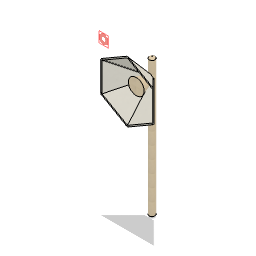
Sarah_meylan (Autodesk Fusion 360 design; units mm, degrees)
Autodesk Fusion 360 part; units mm, degrees
sketch "Esquisse1" plane through (0, 0, 0) normal (0, 1, 0) x (1, 0, 0)
  circle A0 centre (0, 0) radius 16.5
  dimension "d1" = 33
  constraint coincident A0.centre origin
  measures "d1" diameter of A0
extrude "Extrusion1" add sketch "Esquisse1" along normal blind 770 makes body 1
sketch "Esquisse3" plane through (0, 0, 0) normal (0, 1, 0) x (1, 0, 0)
  circle A0 centre (0, 0) radius 14
  dimension "d5" = 28
  constraint coincident A0.centre origin
  measures "d5" diameter of A0
extrude "Extrusion2" cut sketch "Esquisse3" along normal blind 770 bodies 1
sketch "Esquisse4" plane through (0, 0, 0) normal (0, 1, 0) x (1, 0, 0)
  circle A0 centre (0, 0) radius 16.5
  dimension "d8" = 33
  constraint coincident A0.centre origin
  measures "d8" diameter of A0
extrude "Extrusion3" add sketch "Esquisse4" against normal blind 10 separate body makes body 2
fillet "Congé1" radius 15 1 edges at (-15.3834, -10, -5.9667) on bodies 2
sketch "Esquisse6" plane through (0, 0, 0) normal (0, 0, 1) x (1, 0, 0)
sketch "Esquisse7" plane through (0, 0, 0) normal (0, 0, 1) x (1, 0, 0)
  line L0 (-275, 755) -> (-250, 740)
  line L1 (-250, 740) -> (-250, 710)
  line L2 (-250, 710) -> (-275, 695)
  line L3 (-275, 695) -> (-301.8648, 710)
  line L4 (-301.8648, 710) -> (-301.8648, 740)
  line L5 (-301.8648, 740) -> (-275, 755)
  constraint vertical L1
  constraint parallel L1 L4
sketch "Esquisse8" plane through (0, 0, 0) normal (0, 0, 1) x (1, 0, 0)
  line L0 (-275.4763, 755.2472) -> (-302.1986, 739.7984)
  line L1 (-302.1986, 739.7984) -> (-302.1986, 710)
  line L2 (-302.1986, 710) -> (-275.4763, 694.7044)
  line L3 (-275.4763, 694.7044) -> (-249.0191, 710)
  line L4 (-249.0191, 710) -> (-249.0191, 740)
  line L5 (-249.0191, 740) -> (-275.4763, 755.2472)
  constraint vertical L1
  constraint parallel L0 L3
  constraint parallel L1 L4
extrude "Extrusion5" add sketch "Esquisse8" along normal blind 125 draft 45 separate body makes body 3
move_body "Déplacer1" bodies 3 to x (1, 0, 0) y (0, 1, 0) z (0, 0, 1) at (275, -50, 15)
shell "Coque1" thickness 5 removed faces 1 at (-50.9798, 703.9976, 140) on bodies 3
fillet "Congé2" radius 15 tangency weight 2 6 edges at (88.4809, 726.1173, 77.5) (-0.5257, 777.4116, 77.5) (88.4809, 623.9398, 77.5) (-89.6986, 725.8586, 77.5) (-89.6986, 623.7601, 77.5) (-0.3209, 572.6013, 77.5) on bodies 3
sketch "Esquisse9" plane through (0, 0, 20) normal (0, 0, 1) x (1, 0, 0)
  line L0 (23.9099, 688.8032) -> (-0.4746, 702.8559)
  line L1 (-0.4746, 702.8559) -> (-25.1275, 688.6034)
  line L2 (-25.1275, 688.6034) -> (-25.1275, 661.2009)
  line L3 (-25.1275, 661.2009) -> (-0.4814, 647.0937)
  line L4 (-0.4814, 647.0937) -> (23.9099, 661.1949)
  line L5 (23.9099, 661.1949) -> (23.9099, 688.8032)
  circle A0 centre (0.3686, 674.9991) radius 22.5
  dimension "d21" = 45
  measures "d21" diameter of A0
sketch "Esquisse10" plane through (0, 0, 20) normal (0, 0, 1) x (1, 0, 0)
  line L0 (23.9099, 688.8032) -> (-0.4746, 702.8559)
  line L1 (-0.4746, 702.8559) -> (-25.1275, 688.6034)
  line L2 (-25.1275, 688.6034) -> (-25.1275, 661.2009)
  line L3 (-25.1275, 661.2009) -> (-0.4814, 647.0937)
  line L4 (-0.4814, 647.0937) -> (23.9099, 661.1949)
  line L5 (23.9099, 661.1949) -> (23.9099, 688.8032)
  circle A0 through (44.9296, 674.9991, 70) (-22.5704, 713.9702, 70) (-22.5704, 636.0279, 70)
  dimension "d24" = 90
extrude "Extrusion7" add sketch "Esquisse10" against normal blind 70 draft -20 contours A0 in plane through (0, 0, 90) normal (0, 0, 1) bodies 3
sketch "Esquisse15" plane through (0, 0, 0) normal (0, 1, 0) x (1, 0, 0)
  circle A0 centre (125, 0) radius 16.5
  dimension "d31" = 33
  measures "d31" diameter of A0
extrude "Extrusion8" add sketch "Esquisse15" along normal blind 10 separate body makes body 4
move_body "Déplacer2" bodies 4 to x (1, 0, 0) y (0, 1, 0) z (0, 0, 1) at (-125, 770, 0)
fillet "Congé3" radius 15 1 faces at (-0.411, 780, -5.2396) on bodies 4
sketch "Esquisse14" plane through (0, 0, 0) normal (0, 1, 0) x (1, 0, 0)
  circle A0 centre (0, 0) radius 16.5
  dimension "d30" = 33
  constraint coincident A0.centre origin
  measures "d30" diameter of A0
sketch "Esquisse11" plane through (0, 0, 0) normal (0, 0, 1) x (1, 0, 0)
sketch "Esquisse12" plane through (0, 0, 0) normal (0, 1, 0) x (1, 0, 0)
  circle A0 centre (0, 0) radius 16.5
  dimension "d28" = 33
  constraint coincident A0.centre origin
  measures "d28" diameter of A0
sketch "Esquisse13" plane through (0, 0, 0) normal (0, 1, 0) x (1, 0, 0)
  circle A0 centre (0, 0) radius 16.5
  dimension "d29" = 33
  constraint coincident A0.centre origin
  measures "d29" diameter of A0
extrude "Extrusion6" [rolled back] along distance 20 taper angle 0
extrude "Extrusion4" [rolled back] along distance -70 taper angle 45
sketch "Esquisse5" plane through (0, 0, 0) normal (0, 1, 0) x (-1, 0, 0)
  circle A0 centre (0, 0) radius 16.5
sketch "Esquisse2" plane through (0, 0, 0) normal (0, 1, 0) x (1, 0, 0)
  circle A0 centre (0, 0) radius 14
  dimension "d2" = 28
  constraint coincident A0.centre origin
  measures "d2" diameter of A0
